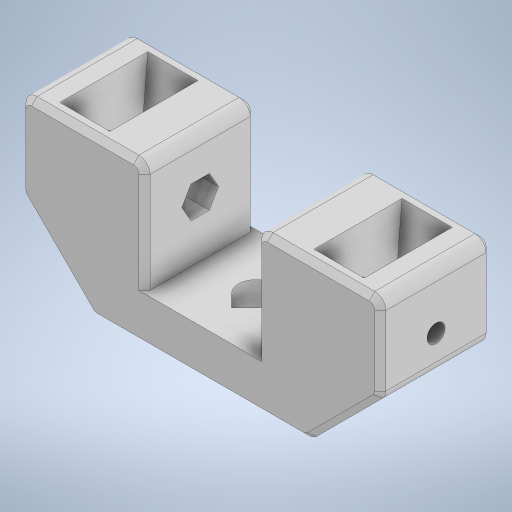
# Autodesk Inventor part: Idle Bearing mount2
Saved by Autodesk Inventor 2023.1 (Build 271208000, 208)
## iProperties
Created: 2022-10-30
Part Number: Idle Bearing mount2
Material: Generic
Document SubType Name: Modeling
Designer: nicol
Density: 1 g/cm^3
Appearance: Default
Author: nicol
Autodesk Inventor part; units mm, degrees
ref_plane "YZ Plane" through (0, 0, 0) normal (1, 0, 0) x (0, 1, 0)
ref_plane "XZ Plane" through (0, 0, 0) normal (0, 1, 0) x (-1, 0, 0)
sketch "Sketch1" plane through (0, 0, 0) normal (0, 0, 1) x (1, 0, 0)
  line L0 (0, 0) -> (0, 28.35)
  line L1 (0, 28.35) -> (8.35, 28.35)
  line L2 (8.35, 28.35) -> (8.35, 8.35)
  line L3 (8.35, 8.35) -> (28.35, 8.35)
  line L4 (28.35, 8.35) -> (28.35, 28.35)
  line L5 (28.35, 28.35) -> (36.7, 28.35)
  line L6 (36.7, 28.35) -> (36.7, 0)
  line L7 (36.7, 0) -> (0, 0)
  dimension "d0" = 20
  dimension "d1" = 8.35
  dimension "d2" = 20
  dimension "d3" = 8.35
  constraints: 16 end point, 7 perpendicular, 2 collinear, 1 vertical
  measures "d0" distance of L2.end L3.end
  measures "d1" distance of L0.end L1.end
  measures "d2" distance of L1.end L2.end
  measures "d3" distance between parallel lines of L7 L3
extrude "Extrusion1" add sketch "Sketch1" along normal blind 20
thicken "Thicken1" operation add thickness 0.05 both sides no extend neighbours yes toward (-1, 0, 0) faces at (8.35, 15.0167, 6.6667) (21.6833, 8.35, 6.6667) (28.35, 21.6833, 6.6667)
sketch "Sketch2" plane through (8.3, 8.3, 0) normal (0, 1, 0) x (1, 0, 0)
  line L0 (20.1, 0) -> (0, 0) projected
  line L1 (0, 0) -> (0, -20) projected
  line L2 (20.1, -20) -> (0, -20) projected
  line L3 (20.1, 0) -> (20.1, -20) projected
  line L4 (10.05, -6.7668) -> (12.85, -8.3834)
  line L5 (12.85, -8.3834) -> (12.85, -11.6166)
  line L6 (12.85, -11.6166) -> (10.05, -13.2332)
  line L7 (10.05, -13.2332) -> (7.25, -11.6166)
  line L8 (7.25, -11.6166) -> (7.25, -8.3834)
  line L9 (7.25, -8.3834) -> (10.05, -6.7668)
  line L10 (0, 0) -> (0, -20) projected
  point P0 (-8.3, 0)
  point P1 (10.05, -10)
  point P2 (0, -10)
  point P3 (10.05, -20)
  dimension "d8" = 5.6
  constraints: 12 end point, 2 midpoint, 1 horizontal alignment, 1 vertical, 1 vertical alignment, 13 other
  measures "d8" distance between parallel lines of L5 L8
hole "Hole1" at (18.35, 8.3, 10) direction (0, -1, 0) diameter 6.2 end through all
sketch "Sketch3" plane through (28.4, 8.3, 0) normal (-1, 0, 0) x (0, 0, 1)
  line L0 (0, 20.05) -> (0, 0) projected
  line L1 (0, 0) -> (20, 0) projected
  line L2 (20, 20.05) -> (20, 0) projected
  line L3 (0, 20.05) -> (20, 20.05) projected
  line L4 (6.7091, 10.025) -> (8.3546, 12.875)
  line L5 (8.3546, 12.875) -> (11.6454, 12.875)
  line L6 (11.6454, 12.875) -> (13.2909, 10.025)
  line L7 (13.2909, 10.025) -> (11.6454, 7.175)
  line L8 (11.6454, 7.175) -> (8.3546, 7.175)
  line L9 (8.3546, 7.175) -> (6.7091, 10.025)
  point P0 (0, -8.3)
  point P1 (10, 10.025)
  point P2 (10, 20.05)
  point P3 (20, 10.025)
  dimension "d19" = 5.7
  constraints: 12 end point, 2 midpoint, 1 horizontal, 1 horizontal alignment, 1 vertical alignment, 13 other
  measures "d19" distance between parallel lines of L6 L9
extrude "Extrusion3" cut sketch "Sketch3" against normal blind 5 contours L4 L5 L6 L7 L8 L9
hole "Hole2" at (28.4, 18.325, 10) direction (1, 0, 0) diameter 3.2 end through all
ref_plane "Work Plane1" through (18.35, 8.3, 0) normal (1, 0, 0) x (0, 0, -1)
sketch "Sketch6" plane through (36.7, 0, 0) normal (1, 0, 0) x (0, 0, -1)
  circle A0 centre (-10, 18.325) radius 1.6 projected
  circle A1 centre (-10, 18.325) radius 7
  line L0 (-3.0266, 17.7149) -> (-2.0962, 28.35)
  line L1 (-16.9734, 17.7149) -> (-17.9038, 28.35)
  line L2 (0, 28.35) -> (-20, 28.35) projected
  circle A2 centre (-10, 18.325) radius 1.6 projected
  line L3 (0, 0) -> (0, 28.35) projected
  line L4 (0, 28.35) -> (-20, 28.35) projected
  line L5 (-20, 0) -> (-20, 28.35) projected
  line L6 (0, 0) -> (-20, 0) projected
  dimension "d47" = 14
  dimension "d48" = 10
  constraints: 4 end point, 2 point on circle, 2 point on line, 2 tangent, 1 centre point, 1 coincident, 1 equal length
  measures "d47" diameter of A1
  measures "d48" angle of L0 L1
extrude "Extrusion6" add sketch "Sketch6" along normal blind 9 contours A1 L0 L2 L3 L6 L5 L1
sketch "Sketch7" plane through (45.7, 0, 0) normal (1, 0, 0) x (0, 0, -1)
  line L0 (-20, 0) -> (0, 0) projected
  line L1 (0, 0) -> (0, 28.35) projected
  line L2 (0, 28.35) -> (-2.0962, 28.35) projected
  line L3 (-2.0962, 28.35) -> (-3.0266, 17.7149) projected
  arc A0 (-16.9734, 17.7149) -> (-3.0266, 17.7149) centre (-10, 18.325) ccw projected
  line L4 (-16.9734, 17.7149) -> (-17.9038, 28.35) projected
  line L5 (-17.9038, 28.35) -> (-20, 28.35) projected
  line L6 (-20, 28.35) -> (-20, 0) projected
  line L7 (-17.9038, 28.35) -> (-2.0962, 28.35)
  line L8 (0, 28.35) -> (-20, 28.35) projected
  circle A1 centre (-10, 18.325) radius 1.6 projected
  constraints: 2 end point, 1 collinear
extrude "Extrusion7" add sketch "Sketch7" along normal blind 5
mirror "Mirror1" about plane through (18.35, 8.3, 0) normal (1, 0, 0) of "Extrusion3", "Hole2", "Extrusion6", "Extrusion7"
chamfer "Chamfer6" distance 13 angle 45 2 edges at (-14, 0, 10) (50.7, 0, 10)
fillet "Fillet3" radius 2 8 edges at (50.7, 28.35, 10) (28.4, 28.35, 10) (8.3, 28.35, 10) (-14, 28.35, 10) (50.7, 13, 10) (37.7, 0, 10) (-1, 0, 10) (-14, 13, 10)
chamfer "Chamfer5" distance 1 angle 45 34 edges at (-14, 20.0892, 20) (-13.8478, 13.0631, 20) (-7.5, 6.5, 20) (-0.9369, 0.1522, 20) (18.35, 0, 20) (37.6369, 0.1522, 20) (44.2, 6.5, 20) (50.5478, 13.0631, 20) (50.7, 20.0892, 20) (50.1142, 27.7642, 20) (39.55, 28.35, 20) (28.9858, 27.7642, 20) (28.4, 17.325, 20) (-13.4142, 27.7642, 20) (-2.85, 28.35, 20) (7.7142, 27.7642, 20) (8.3, 17.325, 20) (-14, 20.0892, 0) (-13.4142, 27.7642, 0) (-2.85, 28.35, 0) (7.7142, 27.7642, 0) (8.3, 17.325, 0) (-13.8478, 13.0631, 0) (-7.5, 6.5, 0) (-0.9369, 0.1522, 0) (18.35, 0, 0) (37.6369, 0.1522, 0) (44.2, 6.5, 0) (50.5478, 13.0631, 0) (50.7, 20.0892, 0) (50.1142, 27.7642, 0) (39.55, 28.35, 0) (28.9858, 27.7642, 0) (28.4, 17.325, 0)
sketch "Sketch8" plane through (-12, 0, 1) normal (0, -1, 0) x (1, 0, 0)
  line L0 (48.8716, 0) -> (11.8284, 0) projected
  line L1 (11.8284, 18) -> (48.8716, 18) projected
  circle A0 centre (30.35, 9) radius 3.1 projected
  line L2 (30.35, 4.6159) -> (34.7341, 9)
  line L3 (34.7341, 9) -> (30.35, 13.3841)
  line L4 (30.35, 13.3841) -> (25.9659, 9)
  line L5 (25.9659, 9) -> (30.35, 4.6159)
  line L6 (30.35, 4.6159) -> (30.35, 13.3841) construction
  line L7 (34.7341, 9) -> (25.9659, 9) construction
  circle A1 centre (30.35, 9) radius 3.1 projected
  line L8 (48.8716, 18) -> (48.8716, 0) projected
  line L9 (11.8284, 0) -> (11.8284, 18) projected
  point P0 (12, -1)
  point P1 (28.158, 11.192)
  point P2 (32.542, 11.192)
  constraints: 12 end point, 2 midpoint, 2 parallel, 2 tangent, 1 perpendicular, 1 vertical
extrude "Extrusion8" cut sketch "Sketch8" against normal through all contours A0 L4 L3
equation "\"d3\" = d1"
body "Solid1"
